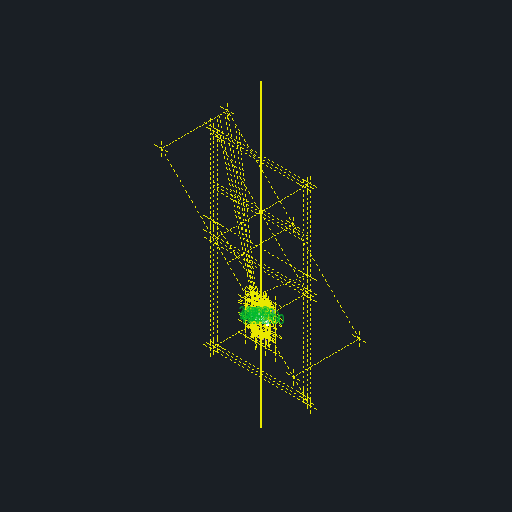
# Autodesk Inventor part: sensorbase
Saved by Autodesk Inventor 2023.5 (Build 275446000, 446)
## iProperties
Created: 2025-01-21
Part Number: sensorbase
Material: 一般
Document SubType Name: Modeling
Designer: IshiiLabHonda
Density: 1 g/cm^3
Appearance: 既定
Author: IshiiLabHonda
Autodesk Inventor part; units mm, degrees
ref_plane "YZ Plane" through (0, 0, 0) normal (1, 0, 0) x (0, 1, 0)
ref_plane "XZ Plane" through (0, 0, 0) normal (0, 1, 0) x (-1, 0, 0)
ref_plane "XY Plane" through (0, 0, 0) normal (0, 0, 1) x (1, 0, 0)
derived "chassis.ipt"
sketch "スケッチ1" plane through (0, 0, 0) normal (0, 0, 1) x (1, 0, 0)
  line L0 (-90, 90) -> (90, 90) construction
  line L1 (90, 90) -> (90, -90) construction
  line L2 (90, -90) -> (-90, -90) construction
  line L3 (-90, -90) -> (-90, 90) construction
  line L4 (-90, 90) -> (-90, 270) construction
  line L5 (-90, 270) -> (90, 270) construction
  line L6 (90, 270) -> (90, 90) construction
  line L7 (-90, 90) -> (90, -90) construction
  line L8 (90, 90) -> (-90, -90) construction
  line L9 (0, 0) -> (0, 10) construction
  line L10 (0, 0) -> (10, 0) construction
  line L11 (-90, 270) -> (90, 90) construction
  line L12 (-90, 90) -> (90, 270) construction
  line L13 (-96, 276) -> (96, 276) construction
  line L14 (96, 276) -> (96, -96) construction
  line L15 (96, -96) -> (-96, -96) construction
  line L16 (-96, -96) -> (-96, 276) construction
  line L17 (-84, 264) -> (84, 264) construction
  line L18 (84, 264) -> (84, -84) construction
  line L19 (84, -84) -> (-84, -84) construction
  line L20 (-84, -84) -> (-84, 264) construction
  line L21 (-96, 96) -> (96, 96) construction
  line L22 (-96, 84) -> (96, 84) construction
  line L23 (-63.6396, 63.6396) -> (63.6396, 190.9188) construction
  line L24 (63.6396, 190.9188) -> (190.9188, 63.6396) construction
  line L25 (190.9188, 63.6396) -> (63.6396, -63.6396) construction
  line L26 (63.6396, -63.6396) -> (-63.6396, 63.6396) construction
  line L27 (-190.9188, 190.9188) -> (-63.6396, 318.1981) construction
  line L28 (-63.6396, 318.1981) -> (63.6396, 190.9188) construction
  line L29 (-63.6396, 63.6396) -> (-190.9188, 190.9188) construction
  line L30 (-96, 120) -> (96, 120) construction
  line L31 (-96, 186) -> (96, 186) construction
  line L32 (-96, 174) -> (96, 174) construction
  line L33 (-96, 180) -> (96, 180) construction
  point P0 (-63.6396, 318.1981)
  point P1 (-90, 120)
  point P2 (90, 120)
  point P3 (0, 180)
sketch "スケッチ2" plane through (0, 0, 0) normal (0, 0, 1) x (1, 0, 0)
  line L0 (63.6396, 190.9188) -> (190.9188, 63.6396) construction
  line L1 (-63.6396, 318.1981) -> (63.6396, 190.9188) construction
  line L2 (-84, 264) -> (84, 264) construction
  line L3 (-90, 270) -> (90, 270) construction
  line L4 (90, 270) -> (90, 90) construction
  line L5 (-96, 276) -> (96, 276) construction
  line L6 (-90, 90) -> (90, 270) construction
  line L7 (-90, 270) -> (90, 90) construction
  line L8 (-63.6396, 63.6396) -> (63.6396, 190.9188) construction
  line L9 (-96, 120) -> (96, 120) construction
  line L10 (-90, 90) -> (90, 90) construction
  line L11 (-96, 96) -> (96, 96) construction
  line L12 (-96, 84) -> (96, 84) construction
  line L13 (90, -90) -> (-90, -90) construction
  line L14 (0, 0) -> (0, 10) construction
  line L15 (0, 0) -> (10, 0) construction
  line L16 (190.9188, 63.6396) -> (63.6396, -63.6396) construction
  line L17 (63.6396, -63.6396) -> (-63.6396, 63.6396) construction
  line L18 (84, -84) -> (-84, -84) construction
  line L19 (96, -96) -> (-96, -96) construction
  line L20 (-90, 90) -> (-90, 270) construction
  line L21 (-63.6396, 63.6396) -> (-190.9188, 190.9188) construction
  line L22 (-190.9188, 190.9188) -> (-63.6396, 318.1981) construction
  line L23 (96, 276) -> (96, -96) construction
  line L24 (-96, -96) -> (-96, 276) construction
  line L25 (84, 264) -> (84, -84) construction
  line L26 (-84, -84) -> (-84, 264) construction
  line L27 (90, 90) -> (90, -90) construction
  line L28 (-90, 90) -> (90, -90) construction
  line L29 (90, 90) -> (-90, -90) construction
  line L30 (-90, -90) -> (-90, 90) construction
  circle A0 centre (0, 0) radius 16.5 construction
  circle A1 centre (0, 0) radius 10 construction
  line L31 (20, 11.5) -> (28.75, 11.5) construction
  line L32 (28.75, 11.5) -> (28.75, -11.5) construction
  line L33 (28.75, -11.5) -> (20, -11.5) construction
  line L34 (20, -11.5) -> (20, 11.5) construction
  line L35 (20, 11.5) -> (18, 11.5) construction
  line L36 (18, 11.5) -> (18, -11.5) construction
  line L37 (18, -11.5) -> (20, -11.5) construction
  line L38 (18, 1.5) -> (17, 1.5) construction
  line L39 (17, -1.5) -> (18, -1.5) construction
  line L40 (-17, 24) -> (17, 24) construction
  line L41 (17, 24) -> (17, -24) construction
  line L42 (17, -24) -> (-17, -24) construction
  line L43 (-17, -24) -> (-17, 24) construction
  line L44 (-20, 11.5) -> (-18, 11.5) construction
  line L45 (-17, -1.5) -> (-18, -1.5) construction
  line L46 (-20, -11.5) -> (-20, 11.5) construction
  line L47 (-18, 11.5) -> (-18, -11.5) construction
  line L48 (-28.75, -11.5) -> (-20, -11.5) construction
  line L49 (-20, 11.5) -> (-28.75, 11.5) construction
  line L50 (-28.75, 11.5) -> (-28.75, -11.5) construction
  line L51 (-18, -11.5) -> (-20, -11.5) construction
  line L52 (-18, 1.5) -> (-17, 1.5) construction
  line L53 (-14.5, 24) -> (-14.5, -24) construction
  line L54 (14.5, 24) -> (14.5, -24) construction
  line L55 (-10.5, 24) -> (-10.5, 19) construction
  line L56 (-10.5, 19) -> (-14.5, 19) construction
  line L57 (-14.5, 24) -> (-10.5, 19) construction
  line L58 (-10.5, 24) -> (-14.5, 19) construction
  circle A2 centre (-12.5, 21.5) radius 1 construction
  line L59 (10.5, 24) -> (10.5, 19) construction
  line L60 (10.5, 19) -> (14.5, 19) construction
  line L61 (10.5, 24) -> (14.5, 19) construction
  line L62 (10.5, 19) -> (14.5, 24) construction
  circle A3 centre (12.5, 21.5) radius 1 construction
  line L63 (-14.5, -19) -> (-10.5, -19) construction
  line L64 (-10.5, -19) -> (-10.5, -24) construction
  line L65 (10.5, -24) -> (10.5, -19) construction
  line L66 (10.5, -19) -> (14.5, -19) construction
  line L67 (-14.5, -19) -> (-10.5, -24) construction
  line L68 (-10.5, -19) -> (-14.5, -24) construction
  circle A4 centre (-12.5, -21.5) radius 1 construction
  line L69 (10.5, -19) -> (14.5, -24) construction
  line L70 (14.5, -19) -> (10.5, -24) construction
  circle A5 centre (12.5, -21.5) radius 1 construction
  point P0 (90, 120)
  point P1 (-90, 120)
  point P2 (-63.6396, 318.1981)
  point P3 (-12.5, -21.5)
  point P4 (-12.5, 21.5)
sketch "スケッチ3" plane through (0, 0, 0) normal (0, 0, 1) x (1, 0, 0)
  line L0 (63.6396, 190.9188) -> (190.9188, 63.6396) construction
  line L1 (-63.6396, 318.1981) -> (63.6396, 190.9188) construction
  line L2 (-84, 264) -> (84, 264) construction
  line L3 (-90, 270) -> (90, 270) construction
  line L4 (90, 270) -> (90, 90) construction
  line L5 (-96, 276) -> (96, 276) construction
  line L6 (-90, 90) -> (90, 270) construction
  line L7 (-90, 270) -> (90, 90) construction
  line L8 (-63.6396, 63.6396) -> (63.6396, 190.9188) construction
  line L9 (-96, 120) -> (96, 120) construction
  line L10 (-90, 90) -> (90, 90) construction
  line L11 (-96, 96) -> (96, 96) construction
  line L12 (-96, 84) -> (96, 84) construction
  line L13 (90, -90) -> (-90, -90) construction
  line L14 (0, 0) -> (0, 10) construction
  line L15 (0, 0) -> (10, 0) construction
  line L16 (190.9188, 63.6396) -> (63.6396, -63.6396) construction
  line L17 (63.6396, -63.6396) -> (-63.6396, 63.6396) construction
  line L18 (84, -84) -> (-84, -84) construction
  line L19 (96, -96) -> (-96, -96) construction
  line L20 (-90, 90) -> (-90, 270) construction
  line L21 (-63.6396, 63.6396) -> (-190.9188, 190.9188) construction
  line L22 (-190.9188, 190.9188) -> (-63.6396, 318.1981) construction
  line L23 (96, 276) -> (96, -96) construction
  line L24 (-96, -96) -> (-96, 276) construction
  line L25 (84, 264) -> (84, -84) construction
  line L26 (-84, -84) -> (-84, 264) construction
  line L27 (90, 90) -> (90, -90) construction
  line L28 (-90, 90) -> (90, -90) construction
  line L29 (90, 90) -> (-90, -90) construction
  line L30 (-90, -90) -> (-90, 90) construction
  line L31 (-18, 1.5) -> (-17, 1.5) construction
  line L32 (-17, -1.5) -> (-18, -1.5) construction
  line L33 (-20, 11.5) -> (-18, 11.5) construction
  line L34 (-28.75, 11.5) -> (-28.75, -11.5) construction
  line L35 (63.6396, -63.6396) -> (-63.6396, 63.6396) construction
  line L36 (84, -84) -> (-84, -84) construction
  line L37 (-90, -90) -> (-90, 90) construction
  line L38 (96, -96) -> (-96, -96) construction
  line L39 (-90, 90) -> (90, 90) construction
  line L40 (90, -90) -> (-90, -90) construction
  line L41 (90, 90) -> (-90, -90) construction
  line L42 (-90, 90) -> (90, -90) construction
  line L43 (90, 90) -> (90, -90) construction
  line L44 (-28.75, -11.5) -> (-20, -11.5) construction
  line L45 (-20, 11.5) -> (-28.75, 11.5) construction
  line L46 (-18, 11.5) -> (-18, -11.5) construction
  line L47 (-18, -11.5) -> (-20, -11.5) construction
  line L48 (0, 0) -> (0, 10) construction
  line L49 (0, 0) -> (10, 0) construction
  circle A0 centre (0, 0) radius 16.5 construction
  circle A1 centre (0, 0) radius 10 construction
  line L50 (-14.5, 24) -> (-14.5, -24) construction
  line L51 (-17, 24) -> (17, 24) construction
  line L52 (-17, -24) -> (-17, 24) construction
  line L53 (17, -24) -> (-17, -24) construction
  line L54 (-14.5, -19) -> (-10.5, -19) construction
  circle A2 centre (-12.5, -21.5) radius 1 construction
  line L55 (-10.5, -19) -> (-14.5, -24) construction
  line L56 (-14.5, -19) -> (-10.5, -24) construction
  line L57 (-63.6396, 318.1981) -> (63.6396, 190.9188) construction
  line L58 (-84, 264) -> (84, 264) construction
  line L59 (-90, 270) -> (90, 270) construction
  line L60 (90, 270) -> (90, 90) construction
  line L61 (-96, 276) -> (96, 276) construction
  line L62 (-90, 90) -> (90, 270) construction
  line L63 (-90, 270) -> (90, 90) construction
  line L64 (-63.6396, 63.6396) -> (63.6396, 190.9188) construction
  line L65 (-96, 120) -> (96, 120) construction
  line L66 (-96, 96) -> (96, 96) construction
  line L67 (-96, 84) -> (96, 84) construction
  line L68 (84, 264) -> (84, -84) construction
  line L69 (96, 276) -> (96, -96) construction
  line L70 (-96, -96) -> (-96, 276) construction
  line L71 (-84, -84) -> (-84, 264) construction
  line L72 (-63.6396, 63.6396) -> (-190.9188, 190.9188) construction
  line L73 (-90, 90) -> (-90, 270) construction
  line L74 (-190.9188, 190.9188) -> (-63.6396, 318.1981) construction
  line L75 (-20, -11.5) -> (-20, 11.5) construction
  line L76 (10.5, -19) -> (14.5, -19) construction
  line L77 (10.5, -24) -> (10.5, -19) construction
  circle A3 centre (12.5, -21.5) radius 1 construction
  line L78 (10.5, -19) -> (14.5, -24) construction
  line L79 (14.5, -19) -> (10.5, -24) construction
  line L80 (-10.5, -19) -> (-10.5, -24) construction
  line L81 (63.6396, 190.9188) -> (190.9188, 63.6396) construction
  line L82 (190.9188, 63.6396) -> (63.6396, -63.6396) construction
  line L83 (20, 11.5) -> (28.75, 11.5) construction
  line L84 (28.75, 11.5) -> (28.75, -11.5) construction
  line L85 (17, -1.5) -> (18, -1.5) construction
  line L86 (18, -11.5) -> (20, -11.5) construction
  line L87 (28.75, -11.5) -> (20, -11.5) construction
  line L88 (14.5, 24) -> (14.5, -24) construction
  line L89 (17, 24) -> (17, -24) construction
  line L90 (18, 11.5) -> (18, -11.5) construction
  line L91 (20, -11.5) -> (20, 11.5) construction
  line L92 (20, 11.5) -> (18, 11.5) construction
  line L93 (18, 1.5) -> (17, 1.5) construction
  line L94 (-10.5, 24) -> (-10.5, 19) construction
  line L95 (10.5, 19) -> (14.5, 19) construction
  circle A4 centre (12.5, 21.5) radius 1 construction
  line L96 (10.5, 24) -> (14.5, 19) construction
  line L97 (10.5, 19) -> (14.5, 24) construction
  line L98 (10.5, 24) -> (10.5, 19) construction
  line L99 (-10.5, 19) -> (-14.5, 19) construction
  circle A5 centre (-12.5, 21.5) radius 1 construction
  line L100 (-14.5, 24) -> (-10.5, 19) construction
  line L101 (-10.5, 24) -> (-14.5, 19) construction
  line L102 (29.25, 41.5) -> (29.25, -41.5) construction
  line L103 (-29.25, -41.5) -> (-29.25, 41.5) construction
  line L104 (-29.25, 8.5) -> (-17, 8.5) construction
  line L105 (-17, 8.5) -> (-17, -8.5) construction
  line L106 (-17, -8.5) -> (-29.25, -8.5) construction
  line L107 (29.25, 8.5) -> (17, 8.5) construction
  line L108 (17, 8.5) -> (17, -8.5) construction
  line L109 (17, -8.5) -> (29.25, -8.5) construction
  line L110 (-2.7087, 12.8503) -> (-1.1893, 4.2332) construction
  line L111 (6.7279, 35.5721) -> (9.9419, 39.4023) construction
  line L112 (5.5106, 35.2882) -> (10.0101, 40.6505) construction
  line L113 (10.4899, 31.11) -> (5.5106, 35.2882) construction
  line L114 (10.0101, 40.6505) -> (10.4899, 31.11) construction
  line L115 (10.5581, 32.3582) -> (9.9419, 39.4023) construction
  line L116 (10.5581, 32.3582) -> (6.7279, 35.5721) construction
  line L117 (10.4899, 31.11) -> (12.788, 29.1817) construction
  line L118 (9.9419, 39.4023) -> (13.7721, 36.1884) construction
  line L119 (6.7279, 35.5721) -> (13.7721, 36.1884) construction
  line L120 (13.7721, 36.1884) -> (10.5581, 32.3582) construction
  line L121 (5.5106, 35.2882) -> (14.9894, 36.4724) construction
  line L122 (10.0101, 40.6505) -> (14.9894, 36.4724) construction
  line L123 (14.9894, 36.4724) -> (10.4899, 31.11) construction
  line L124 (12.788, 29.1817) -> (17.2875, 34.544) construction
  line L125 (17.2875, 34.544) -> (14.9894, 36.4724) construction
  line L126 (-3.5633, 11.938) -> (-2.695, 7.014) construction
  line L127 (-8.4873, 11.0698) -> (-2.695, 7.014) construction
  line L128 (-7.6191, 6.1457) -> (-3.5633, 11.938) construction
  line L129 (-9.1099, 11.7216) -> (-2.7087, 12.8503) construction
  line L130 (-7.6191, 6.1457) -> (-8.4873, 11.0698) construction
  line L131 (-1.1893, 4.2332) -> (-7.5905, 3.1045) construction
  line L132 (-63.6396, 318.1981) -> (-5.5912, 9.0419) construction
  line L133 (10.25, 35.8803) -> (-90, 120) construction
  line L134 (-5.5912, 9.0419) -> (-79.4589, 302.3788) construction
  line L135 (-5.5912, 9.0419) -> (-41.5175, 296.076) construction
  line L136 (-10.25, 35.8803) -> (90, 120) construction
  line L137 (-9.9419, 39.4023) -> (-6.7279, 35.5721) construction
  line L138 (-10.0101, 40.6505) -> (-5.5106, 35.2882) construction
  line L139 (-14.9894, 36.4724) -> (-10.0101, 40.6505) construction
  line L140 (-5.5106, 35.2882) -> (-14.9894, 36.4724) construction
  line L141 (-13.7721, 36.1884) -> (-6.7279, 35.5721) construction
  line L142 (-13.7721, 36.1884) -> (-9.9419, 39.4023) construction
  line L143 (-14.9894, 36.4724) -> (-17.2875, 34.544) construction
  line L144 (-6.7279, 35.5721) -> (-10.5581, 32.3582) construction
  line L145 (-9.9419, 39.4023) -> (-10.5581, 32.3582) construction
  line L146 (-10.0101, 40.6505) -> (-10.4899, 31.11) construction
  line L147 (-5.5106, 35.2882) -> (-10.4899, 31.11) construction
  line L148 (-10.4899, 31.11) -> (-14.9894, 36.4724) construction
  line L149 (-17.2875, 34.544) -> (-12.788, 29.1817) construction
  line L150 (-12.788, 29.1817) -> (-10.4899, 31.11) construction
  line L151 (-10.5581, 32.3582) -> (-13.7721, 36.1884) construction
  circle A6 centre (-7.0361, 32.05) radius 0.625 construction
  circle A7 centre (-7.0361, 32.05) radius 0.8 construction
  circle A8 centre (-7.0361, 32.05) radius 1.5 construction
  circle A9 centre (-16.0715, 34.6506) radius 1.5 construction
  circle A10 centre (-16.0715, 34.6506) radius 0.8 construction
  circle A11 centre (-16.0715, 34.6506) radius 0.625 construction
  line L152 (-2.695, 7.014) -> (-7.6191, 6.1457) construction
  line L153 (-7.9812, 5.3203) -> (-1.58, 6.449) construction
  line L154 (-8.0532, 8.6078) -> (-3.1291, 9.476) construction
  line L155 (-4.6361, 3.6254) -> (-5.157, 6.5799) construction
  line L156 (-8.4873, 11.0698) -> (-3.5633, 11.938) construction
  circle A12 centre (16.0715, 34.6506) radius 1.5 construction
  circle A13 centre (16.0715, 34.6506) radius 0.625 construction
  circle A14 centre (16.0715, 34.6506) radius 0.8 construction
  circle A15 centre (7.0361, 32.05) radius 1.5 construction
  circle A16 centre (7.0361, 32.05) radius 0.8 construction
  circle A17 centre (7.0361, 32.05) radius 0.625 construction
  line L157 (-29.25, -41.5) -> (29.25, -41.5) construction
  line L158 (-29.25, 41.5) -> (29.25, 41.5) construction
  line L159 (-10.25, 35.8803) -> (-7.0361, 32.05) construction
  line L160 (-29.25, 20.8653) -> (-13.3068, 41.5) construction
  line L161 (-29.25, -21.1569) -> (-8.9069, -41.5) construction
  line L162 (29.25, 20.8653) -> (13.3068, 41.5) construction
  line L163 (29.25, -21.1569) -> (8.9069, -41.5) construction
  line L164 (25.25, 19.5) -> (25.25, 14.5) construction
  line L165 (25.25, 14.5) -> (17, 14.5) construction
  line L166 (4.1128, 32.222) -> (-2.9985, 32.8014) construction
  line L167 (-17, 14.5) -> (-25.25, 14.5) construction
  line L168 (-25.25, 14.5) -> (-25.25, 19.5) construction
  line L169 (1.1893, 4.2332) -> (7.5905, 3.1045) construction
  line L170 (7.5905, 3.1045) -> (9.1099, 11.7216) construction
  line L171 (2.7087, 12.8503) -> (1.1893, 4.2332) construction
  line L172 (2.695, 7.014) -> (7.6191, 6.1457) construction
  line L173 (7.9812, 5.3203) -> (1.58, 6.449) construction
  line L174 (8.4873, 11.0698) -> (2.695, 7.014) construction
  line L175 (7.6191, 6.1457) -> (3.5633, 11.938) construction
  line L176 (3.5633, 11.938) -> (2.695, 7.014) construction
  line L177 (8.4873, 11.0698) -> (3.5633, 11.938) construction
  line L178 (7.6191, 6.1457) -> (8.4873, 11.0698) construction
  line L179 (9.1099, 11.7216) -> (2.7087, 12.8503) construction
  line L180 (-13.5, 30.3157) -> (-13.5, 24) construction
  line L181 (13.5, 30) -> (13.5, 24) construction
  line L182 (13.5, 24) -> (17, 24) construction
  line L183 (17, 24) -> (17, 14.5) construction
  line L184 (-13.5, 24) -> (-17, 24) construction
  line L185 (-17, 24) -> (-17, 14.5) construction
  line L186 (-13.5, 30.3157) -> (-2.9985, 32.8014) construction
  line L187 (13.5, 30) -> (4.1128, 32.222) construction
  line L188 (-17, -14.5) -> (-25.25, -14.5) construction
  line L189 (-25.25, -14.5) -> (-25.25, -19.5) construction
  line L190 (-25.25, -19.5) -> (-7.25, -37.5) construction
  line L191 (-7.25, -37.5) -> (7.25, -37.5) construction
  line L192 (7.25, -37.5) -> (25.25, -19.5) construction
  line L193 (25.25, -19.5) -> (25.25, -14.5) construction
  line L194 (25.25, -14.5) -> (17, -14.5) construction
  line L195 (17, -14.5) -> (17, -24) construction
  line L196 (17, -24) -> (13.5, -24) construction
  line L197 (13.5, -24) -> (11.356, -30.1704) construction
  line L198 (11.356, -30.1704) -> (-13.5, -30) construction
  line L199 (-13.5, -30) -> (-13.5, -24) construction
  line L200 (-13.5, -24) -> (-17, -24) construction
  line L201 (-17, -24) -> (-17, -14.5) construction
  line L202 (-9.1099, 11.7216) -> (-7.5905, 3.1045) construction
  line L203 (-9.4721, 10.8961) -> (-8.6039, 5.9721) construction
  line L204 (-14.3961, 10.0279) -> (-8.6039, 5.9721) construction
  line L205 (-13.5279, 5.1039) -> (-9.4721, 10.8961) construction
  line L206 (-13.5279, 5.1039) -> (-14.3961, 10.0279) construction
  line L207 (-7.5905, 3.1045) -> (-13.9918, 1.9758) construction
  line L208 (-14.3961, 10.0279) -> (-9.4721, 10.8961) construction
  line L209 (-13.962, 7.5659) -> (-9.038, 8.4341) construction
  line L210 (-8.6039, 5.9721) -> (-13.5279, 5.1039) construction
  line L211 (-10.5449, 2.5836) -> (-11.0659, 5.538) construction
  line L212 (-15.5112, 10.5929) -> (-9.1099, 11.7216) construction
  line L213 (9.4721, 10.8961) -> (8.6039, 5.9721) construction
  line L214 (9.1099, 11.7216) -> (7.5905, 3.1045) construction
  line L215 (14.3961, 10.0279) -> (9.4721, 10.8961) construction
  line L216 (13.962, 7.5659) -> (9.038, 8.4341) construction
  line L217 (10.5449, 2.5836) -> (11.0659, 5.538) construction
  line L218 (15.5112, 10.5929) -> (9.1099, 11.7216) construction
  line L219 (13.5279, 5.1039) -> (9.4721, 10.8961) construction
  line L220 (8.6039, 5.9721) -> (13.5279, 5.1039) construction
  line L221 (14.3961, 10.0279) -> (8.6039, 5.9721) construction
  line L222 (13.5279, 5.1039) -> (14.3961, 10.0279) construction
  line L223 (13.9918, 1.9758) -> (15.5112, 10.5929) construction
  line L224 (7.5905, 3.1045) -> (13.9918, 1.9758) construction
  line L225 (-25.25, 19.5) -> (-11.3425, 37.5) construction
  line L226 (-11.3425, 37.5) -> (11.3425, 37.5) construction
  line L227 (11.3425, 37.5) -> (25.25, 19.5) construction
  circle A18 centre (0, 0) radius 4.25 construction
  line L228 (-11.5, 8) -> (-68.7791, 313.0586) construction
  line L229 (-11.5, 8) -> (-84.3887, 297.449) construction
  line L230 (-11.5, 8) -> (-48.4208, 302.9793) construction
  line L231 (-15.5112, 10.5929) -> (-13.9918, 1.9758) construction
  line L232 (-14.3825, 4.1916) -> (-7.9812, 5.3203) construction
  circle A19 centre (-10.5, -27) radius 1
  circle A20 centre (10.5, 27) radius 1
  circle A21 centre (10.5, 27) radius 2
  circle A22 centre (-10.5, -27) radius 2
  circle A23 centre (0, -27) radius 1
  circle A24 centre (0, -27) radius 2
  circle A25 centre (0, 27) radius 1
  circle A26 centre (0, 27) radius 2
  line L233 (0, 27) -> (10.5, 27) construction
  line L234 (-10.5, -27) -> (0, -27) construction
  line L235 (13.5, 30) -> (-3, 30)
  line L236 (-3, 30) -> (-3, 24)
  line L237 (-13.5, 24) -> (-3, 24)
  line L238 (-13.5, -30) -> (3, -30)
  line L239 (3, -30) -> (3, -24)
  line L240 (3, -24) -> (13.5, -24)
  line L241 (-16.1606, 31.2641) -> (-6.1594, 29.9135)
  line L242 (-6.1594, 29.9135) -> (-5.0634, 31.332)
  line L243 (-5.0634, 31.332) -> (-4.8147, 37.5)
  line L244 (6.1594, 29.9135) -> (5.0634, 31.332)
  line L245 (16.1606, 31.2641) -> (6.1594, 29.9135)
  line L246 (5.0634, 31.332) -> (4.8147, 37.5)
  line L247 (-10.5, -27) -> (-14.125, -30.625) construction
  line L248 (-15.5392, -29.2108) -> (-13.5, -24)
  line L249 (-12.7108, -32.0392) -> (-7.5, -30)
  line L250 (10.5, 27) -> (13.5, 30) construction
  line L251 (16.1606, 31.2641) -> (10.0926, 30)
  line L252 (-10.5, -19) -> (-10.5, -20.4081)
  line L253 (-10.5, -20.4081) -> (-7.5, -21.5)
  line L254 (-7.5, -21.5) -> (7.5, -21.5)
  line L255 (7.5, -21.5) -> (10.5, -20.4081)
  line L256 (10.5, -20.4081) -> (10.5, -19)
  line L257 (10.5, -19) -> (-10.5, -19)
  line L258 (7.5, 21.5) -> (10.5, 20.4081)
  line L259 (10.5, 20.4081) -> (10.5, 19)
  line L260 (-7.5, 21.5) -> (7.5, 21.5)
  line L261 (10.5, 19) -> (-10.5, 19)
  line L262 (-10.5, 19) -> (-10.5, 20.4081)
  line L263 (-10.5, 20.4081) -> (-7.5, 21.5)
  line L264 (-5.3602, -19) -> (-14.5, -13.3971)
  line L265 (-14.5, -13.3971) -> (-14.5, -15.3971)
  line L266 (0, 0) -> (-9.9301, -16.1985) construction
  line L267 (14.5, -13.3971) -> (14.5, -15.3971)
  line L268 (5.3602, -19) -> (14.5, -13.3971)
  line L269 (-5.3602, 19) -> (-14.5, 13.3971)
  line L270 (-14.5, 13.3971) -> (-14.5, 15.3971)
  line L271 (5.3602, 19) -> (14.5, 13.3971)
  line L272 (14.5, 13.3971) -> (14.5, 15.3971)
  line L273 (-14.5, -15.3971) -> (-10.5, -20.4081)
  line L274 (10.5, -20.4081) -> (14.5, -15.3971)
  line L275 (-14.5, 15.3971) -> (-10.5, 20.4081)
  line L276 (14.5, 15.3971) -> (10.5, 20.4081)
  line L277 (-5.3602, -19) -> (-9.4462, -17.5128)
  line L278 (-9.4462, -17.5128) -> (-14.5, -13.3971)
  line L279 (-10.5, -20.4081) -> (-9.4462, -17.5128) construction
  line L280 (9.4462, -17.5128) -> (14.5, -13.3971)
  line L281 (5.3602, -19) -> (9.4462, -17.5128)
  line L282 (-5.3602, 19) -> (-9.4462, 17.5128)
  line L283 (-9.4462, 17.5128) -> (-14.5, 13.3971)
  line L284 (9.4462, 17.5128) -> (14.5, 13.3971)
  line L285 (5.3602, 19) -> (9.4462, 17.5128)
  point P0 (90, 120)
  point P1 (90, 120)
  point P2 (25.25, 25.1515)
  point P3 (11.5, 8)
  point P4 (11.5, 8)
  point P5 (-5.5912, 9.0419)
  point P6 (-5.5912, 9.0419)
  point P7 (13.6038, 24)
  point P8 (6.0926, 30)
sketch "スケッチ4" plane through (0, 0, 0) normal (1, 0, 0) x (0, 1, 0)
  circle A0 centre (15.0669, 9.7) radius 4.35 construction
  line L0 (0, 8.7) -> (0, 9.7) construction
  circle A1 centre (0, 8.7) radius 10.65 construction
  circle A2 centre (0, 8.7) radius 11.5 construction
  line L1 (-25, -2.8) -> (25, -2.8) construction
  line L2 (-25, -1) -> (25, -1) construction
  line L3 (-25, 0) -> (25, 0) construction
  line L4 (0, 8.7) -> (1, 8.7) construction
  circle A3 centre (-13, 8.7) radius 2.25 construction
  line L5 (0, -7.4) -> (0, 24.8)
  line L6 (-178.8396, 0) -> (401.0377, 0)
  point P0 (0, 0)
  point P1 (0, 0)
sketch "スケッチ5" plane through (0, 0, 0) normal (0, 0, 1) x (1, 0, 0)
  line L0 (0, 0) -> (0, 10) construction
  line L1 (0, 0) -> (10, 0) construction
  line L2 (-17, -1.5) -> (-18, -1.5) construction
  line L3 (-28.75, -11.5) -> (-20, -11.5) construction
  line L4 (-18, 1.5) -> (-17, 1.5) construction
  line L5 (-18, 11.5) -> (-18, -11.5) construction
  line L6 (-20, 11.5) -> (-18, 11.5) construction
  line L7 (-20, -11.5) -> (-20, 11.5) construction
  line L8 (-20, 11.5) -> (-28.75, 11.5) construction
  line L9 (-28.75, 11.5) -> (-28.75, -11.5) construction
  line L10 (28.75, 11.5) -> (28.75, -11.5) construction
  line L11 (28.75, -11.5) -> (20, -11.5) construction
  line L12 (20, 11.5) -> (28.75, 11.5) construction
  line L13 (20, 11.5) -> (18, 11.5) construction
  line L14 (18, 1.5) -> (17, 1.5) construction
  line L15 (20, -11.5) -> (20, 11.5) construction
  line L16 (18, -11.5) -> (20, -11.5) construction
  line L17 (18, 11.5) -> (18, -11.5) construction
  circle A0 centre (0, 0) radius 10 construction
  line L18 (17, 24) -> (17, -24) construction
  line L19 (-17, 24) -> (17, 24) construction
  line L20 (14.5, 24) -> (14.5, -24) construction
  circle A1 centre (0, 0) radius 16.5 construction
  line L21 (-14.5, 24) -> (-14.5, -24) construction
  line L22 (-17, -24) -> (-17, 24) construction
  line L23 (17, -24) -> (-17, -24) construction
  line L24 (17, -1.5) -> (18, -1.5) construction
  line L25 (-18, -11.5) -> (-20, -11.5) construction
  line L26 (-10.5, 19) -> (-14.5, 19) construction
  line L27 (-10.5, 24) -> (-10.5, 19) construction
  circle A2 centre (-12.5, 21.5) radius 1 construction
  line L28 (-14.5, 24) -> (-10.5, 19) construction
  line L29 (-10.5, 24) -> (-14.5, 19) construction
  line L30 (10.5, 24) -> (10.5, 19) construction
  circle A3 centre (12.5, 21.5) radius 1 construction
  line L31 (10.5, 24) -> (14.5, 19) construction
  line L32 (10.5, 19) -> (14.5, 24) construction
  line L33 (10.5, 19) -> (14.5, 19) construction
  line L34 (-14.5, -19) -> (-10.5, -19) construction
  circle A4 centre (-12.5, -21.5) radius 1 construction
  line L35 (-14.5, -19) -> (-10.5, -24) construction
  line L36 (-10.5, -19) -> (-14.5, -24) construction
  line L37 (-10.5, -19) -> (-10.5, -24) construction
  line L38 (10.5, -19) -> (14.5, -19) construction
  circle A5 centre (12.5, -21.5) radius 1 construction
  line L39 (10.5, -19) -> (14.5, -24) construction
  line L40 (14.5, -19) -> (10.5, -24) construction
  line L41 (10.5, -24) -> (10.5, -19) construction
  line L42 (13.5, 24) -> (17, 24) construction
  line L43 (4.1128, 32.222) -> (-2.9985, 32.8014) construction
  line L44 (17, 8.5) -> (17, -8.5) construction
  line L45 (10.5449, 2.5836) -> (11.0659, 5.538) construction
  line L46 (13.5279, 5.1039) -> (9.4721, 10.8961) construction
  line L47 (8.6039, 5.9721) -> (13.5279, 5.1039) construction
  line L48 (13.962, 7.5659) -> (9.038, 8.4341) construction
  line L49 (14.3961, 10.0279) -> (9.4721, 10.8961) construction
  line L50 (14.3961, 10.0279) -> (8.6039, 5.9721) construction
  line L51 (13.5279, 5.1039) -> (14.3961, 10.0279) construction
  line L52 (7.5905, 3.1045) -> (13.9918, 1.9758) construction
  line L53 (15.5112, 10.5929) -> (9.1099, 11.7216) construction
  line L54 (13.9918, 1.9758) -> (15.5112, 10.5929) construction
  line L55 (20, 11.5) -> (28.75, 11.5) construction
  line L56 (20, 11.5) -> (18, 11.5) construction
  line L57 (10.5, 19) -> (14.5, 19) construction
  circle A6 centre (12.5, 21.5) radius 1 construction
  line L58 (29.25, 8.5) -> (17, 8.5) construction
  line L59 (13.5, 30) -> (13.5, 24) construction
  line L60 (25.25, 14.5) -> (17, 14.5) construction
  line L61 (25.25, 19.5) -> (25.25, 14.5) construction
  line L62 (13.5, 30) -> (4.1128, 32.222) construction
  line L63 (17, 24) -> (17, 14.5) construction
  line L64 (9.1099, 11.7216) -> (2.7087, 12.8503) construction
  line L65 (8.4873, 11.0698) -> (3.5633, 11.938) construction
  line L66 (-8.4873, 11.0698) -> (-3.5633, 11.938) construction
  line L67 (-17, 8.5) -> (-17, -8.5) construction
  line L68 (-7.6191, 6.1457) -> (-8.4873, 11.0698) construction
  line L69 (-7.5905, 3.1045) -> (-13.9918, 1.9758) construction
  line L70 (-14.3825, 4.1916) -> (-7.9812, 5.3203) construction
  line L71 (-10.5449, 2.5836) -> (-11.0659, 5.538) construction
  line L72 (-8.6039, 5.9721) -> (-13.5279, 5.1039) construction
  line L73 (-13.962, 7.5659) -> (-9.038, 8.4341) construction
  line L74 (-14.3961, 10.0279) -> (-8.6039, 5.9721) construction
  line L75 (-13.5279, 5.1039) -> (-14.3961, 10.0279) construction
  line L76 (-15.5112, 10.5929) -> (-13.9918, 1.9758) construction
  line L77 (-9.4721, 10.8961) -> (-8.6039, 5.9721) construction
  line L78 (-13.5279, 5.1039) -> (-9.4721, 10.8961) construction
  line L79 (-9.1099, 11.7216) -> (-7.5905, 3.1045) construction
  line L80 (-14.3961, 10.0279) -> (-9.4721, 10.8961) construction
  line L81 (-15.5112, 10.5929) -> (-9.1099, 11.7216) construction
  line L82 (2.7087, 12.8503) -> (1.1893, 4.2332) construction
  line L83 (3.5633, 11.938) -> (2.695, 7.014) construction
  line L84 (7.6191, 6.1457) -> (3.5633, 11.938) construction
  line L85 (7.6191, 6.1457) -> (8.4873, 11.0698) construction
  line L86 (2.695, 7.014) -> (7.6191, 6.1457) construction
  line L87 (9.4721, 10.8961) -> (8.6039, 5.9721) construction
  line L88 (7.9812, 5.3203) -> (1.58, 6.449) construction
  line L89 (1.1893, 4.2332) -> (7.5905, 3.1045) construction
  line L90 (7.5905, 3.1045) -> (9.1099, 11.7216) construction
  line L91 (9.1099, 11.7216) -> (7.5905, 3.1045) construction
  line L92 (8.4873, 11.0698) -> (2.695, 7.014) construction
  line L93 (0, 0) -> (0, 10) construction
  circle A7 centre (0, 0) radius 4.25 construction
  line L94 (-2.7087, 12.8503) -> (-1.1893, 4.2332) construction
  line L95 (-3.5633, 11.938) -> (-2.695, 7.014) construction
  line L96 (-4.6361, 3.6254) -> (-5.157, 6.5799) construction
  line L97 (-1.1893, 4.2332) -> (-7.5905, 3.1045) construction
  line L98 (-2.695, 7.014) -> (-7.6191, 6.1457) construction
  line L99 (-7.6191, 6.1457) -> (-3.5633, 11.938) construction
  line L100 (-8.4873, 11.0698) -> (-2.695, 7.014) construction
  line L101 (-7.9812, 5.3203) -> (-1.58, 6.449) construction
  line L102 (-11.3425, 37.5) -> (11.3425, 37.5) construction
  line L103 (-10.25, 35.8803) -> (-7.0361, 32.05) construction
  line L104 (11.3425, 37.5) -> (25.25, 19.5) construction
  line L105 (29.25, 20.8653) -> (13.3068, 41.5) construction
  circle A8 centre (16.0715, 34.6506) radius 1.5 construction
  circle A9 centre (16.0715, 34.6506) radius 0.8 construction
  circle A10 centre (16.0715, 34.6506) radius 0.625 construction
  line L106 (0, 0) -> (0, 10) construction
  line L107 (0, 0) -> (10, 0) construction
  circle A11 centre (0, 0) radius 16.5 construction
  circle A12 centre (0, 0) radius 10 construction
  line L108 (-14.5, 24) -> (-14.5, -24) construction
  line L109 (-17, 24) -> (17, 24) construction
  line L110 (-9.1099, 11.7216) -> (-2.7087, 12.8503) construction
  line L111 (-14.5, -19) -> (-10.5, -19) construction
  circle A13 centre (-12.5, -21.5) radius 1 construction
  line L112 (-17, -24) -> (-17, 24) construction
  line L113 (17, -24) -> (-17, -24) construction
  line L114 (-10.5, -19) -> (-14.5, -24) construction
  line L115 (-14.5, -19) -> (-10.5, -24) construction
  line L116 (-28.75, 11.5) -> (-28.75, -11.5) construction
  line L117 (-9.9419, 39.4023) -> (-6.7279, 35.5721) construction
  line L118 (-10.0101, 40.6505) -> (-5.5106, 35.2882) construction
  line L119 (-13.7721, 36.1884) -> (-6.7279, 35.5721) construction
  line L120 (-5.5106, 35.2882) -> (-14.9894, 36.4724) construction
  line L121 (-13.7721, 36.1884) -> (-9.9419, 39.4023) construction
  line L122 (-14.9894, 36.4724) -> (-10.0101, 40.6505) construction
  line L123 (-14.9894, 36.4724) -> (-17.2875, 34.544) construction
  circle A14 centre (-7.0361, 32.05) radius 0.625 construction
  circle A15 centre (-7.0361, 32.05) radius 0.8 construction
  circle A16 centre (-7.0361, 32.05) radius 1.5 construction
  line L124 (-5.5106, 35.2882) -> (-10.4899, 31.11) construction
  line L125 (-6.7279, 35.5721) -> (-10.5581, 32.3582) construction
  line L126 (-9.9419, 39.4023) -> (-10.5581, 32.3582) construction
  line L127 (-10.0101, 40.6505) -> (-10.4899, 31.11) construction
  line L128 (-12.788, 29.1817) -> (-10.4899, 31.11) construction
  line L129 (-10.5581, 32.3582) -> (-13.7721, 36.1884) construction
  circle A17 centre (-16.0715, 34.6506) radius 0.625 construction
  circle A18 centre (-16.0715, 34.6506) radius 0.8 construction
  circle A19 centre (-16.0715, 34.6506) radius 1.5 construction
  line L130 (-17.2875, 34.544) -> (-12.788, 29.1817) construction
  line L131 (-10.4899, 31.11) -> (-14.9894, 36.4724) construction
  line L132 (-18, 11.5) -> (-18, -11.5) construction
  line L133 (-20, 11.5) -> (-18, 11.5) construction
  line L134 (-10.5, 24) -> (-10.5, 19) construction
  line L135 (-10.5, 19) -> (-14.5, 19) construction
  circle A20 centre (-12.5, 21.5) radius 1 construction
  line L136 (-14.5, 24) -> (-10.5, 19) construction
  line L137 (-10.5, 24) -> (-14.5, 19) construction
  line L138 (-8.0532, 8.6078) -> (-3.1291, 9.476) construction
  line L139 (-17, 14.5) -> (-25.25, 14.5) construction
  line L140 (-25.25, 14.5) -> (-25.25, 19.5) construction
  line L141 (-13.5, 30.3157) -> (-2.9985, 32.8014) construction
  line L142 (-13.5, 30.3157) -> (-13.5, 24) construction
  line L143 (-13.5, 24) -> (-17, 24) construction
  line L144 (-25.25, 19.5) -> (-11.3425, 37.5) construction
  line L145 (-17, 24) -> (-17, 14.5) construction
  line L146 (-17, -24) -> (-17, -14.5) construction
  line L147 (-17, -14.5) -> (-25.25, -14.5) construction
  line L148 (-25.25, -14.5) -> (-25.25, -19.5) construction
  line L149 (-25.25, -19.5) -> (-7.25, -37.5) construction
  line L150 (-29.25, -21.1569) -> (-8.9069, -41.5) construction
  line L151 (10.5, -19) -> (14.5, -19) construction
  line L152 (10.5, -24) -> (10.5, -19) construction
  circle A21 centre (12.5, -21.5) radius 1 construction
  line L153 (10.5, -19) -> (14.5, -24) construction
  line L154 (14.5, -19) -> (10.5, -24) construction
  line L155 (-10.5, -19) -> (-10.5, -24) construction
  line L156 (18, -11.5) -> (20, -11.5) construction
  line L157 (28.75, -11.5) -> (20, -11.5) construction
  line L158 (17, -8.5) -> (29.25, -8.5) construction
  line L159 (-29.25, -41.5) -> (29.25, -41.5) construction
  line L160 (-7.25, -37.5) -> (7.25, -37.5) construction
  line L161 (11.356, -30.1704) -> (-13.5, -30) construction
  line L162 (13.5, -24) -> (11.356, -30.1704) construction
  line L163 (17, -24) -> (13.5, -24) construction
  line L164 (17, -14.5) -> (17, -24) construction
  line L165 (7.25, -37.5) -> (25.25, -19.5) construction
  line L166 (29.25, -21.1569) -> (8.9069, -41.5) construction
  line L167 (25.25, -14.5) -> (17, -14.5) construction
  line L168 (25.25, -19.5) -> (25.25, -14.5) construction
  line L169 (10.0101, 40.6505) -> (14.9894, 36.4724) construction
  line L170 (10.4899, 31.11) -> (12.788, 29.1817) construction
  line L171 (12.788, 29.1817) -> (17.2875, 34.544) construction
  line L172 (17.2875, 34.544) -> (14.9894, 36.4724) construction
  line L173 (-29.25, 41.5) -> (29.25, 41.5) construction
  line L174 (13.7721, 36.1884) -> (10.5581, 32.3582) construction
  line L175 (14.9894, 36.4724) -> (10.4899, 31.11) construction
  circle A22 centre (7.0361, 32.05) radius 0.625 construction
  circle A23 centre (7.0361, 32.05) radius 0.8 construction
  line L176 (10.5581, 32.3582) -> (9.9419, 39.4023) construction
  line L177 (9.9419, 39.4023) -> (13.7721, 36.1884) construction
  circle A24 centre (7.0361, 32.05) radius 1.5 construction
  line L178 (10.5581, 32.3582) -> (6.7279, 35.5721) construction
  line L179 (6.7279, 35.5721) -> (13.7721, 36.1884) construction
  line L180 (5.5106, 35.2882) -> (14.9894, 36.4724) construction
  line L181 (10.0101, 40.6505) -> (10.4899, 31.11) construction
  line L182 (6.7279, 35.5721) -> (9.9419, 39.4023) construction
  line L183 (5.5106, 35.2882) -> (10.0101, 40.6505) construction
  line L184 (10.4899, 31.11) -> (5.5106, 35.2882) construction
  line L185 (-13.5, -24) -> (-17, -24) construction
  line L186 (-13.5, -30) -> (-13.5, -24) construction
  line L187 (-17, -8.5) -> (-29.25, -8.5) construction
  line L188 (-20, -11.5) -> (-20, 11.5) construction
  line L189 (17, -1.5) -> (18, -1.5) construction
  line L190 (18, 1.5) -> (17, 1.5) construction
  line L191 (-29.25, -41.5) -> (-29.25, 41.5) construction
  line L192 (18, 11.5) -> (18, -11.5) construction
  line L193 (20, -11.5) -> (20, 11.5) construction
  line L194 (29.25, 41.5) -> (29.25, -41.5) construction
  line L195 (28.75, 11.5) -> (28.75, -11.5) construction
  line L196 (14.5, 24) -> (14.5, -24) construction
  line L197 (17, 24) -> (17, -24) construction
  line L198 (10.5, 24) -> (14.5, 19) construction
  line L199 (10.5, 19) -> (14.5, 24) construction
  line L200 (10.5, 24) -> (10.5, 19) construction
  line L201 (-20, 11.5) -> (-28.75, 11.5) construction
  line L202 (-28.75, -11.5) -> (-20, -11.5) construction
  line L203 (-18, -11.5) -> (-20, -11.5) construction
  line L204 (-18, 1.5) -> (-17, 1.5) construction
  line L205 (-17, -1.5) -> (-18, -1.5) construction
  line L206 (0, 0) -> (10, 0) construction
  line L207 (-29.25, 20.8653) -> (-13.3068, 41.5) construction
  line L208 (-29.25, 8.5) -> (-17, 8.5) construction
  line L209 (0, 0) -> (0, 10) construction
  line L210 (0, 0) -> (10, 0) construction
  line L211 (0, -10.65) -> (0, 10.65) construction
  line L212 (0, 0) -> (0, 1) construction
  line L213 (0, -15.25) -> (0, -10.75) construction
  line L214 (0, 10.7169) -> (0, 19.4169) construction
  line L215 (0, -11.5) -> (0, 11.5) construction
  line L216 (0, -25) -> (0, 25) construction
  line L217 (0, -25) -> (0, 25) construction
  line L218 (0, -25) -> (0, 25) construction
  circle A25 centre (-12.5, 6) radius 1
  circle A26 centre (-12.5, 6) radius 2.5
  circle A27 centre (-12.5, 6) radius 0.8 construction
  circle A28 centre (12.5, 6) radius 1
  circle A29 centre (12.5, 6) radius 2.5
  circle A30 centre (12.5, 6) radius 0.8 construction
  line L219 (-12.5, 3.5) -> (12.5, 3.5)
  line L220 (-12.5, 8.5) -> (12.5, 8.5)
  line L221 (-3.499, 11) -> (3.499, 11)
  line L222 (3.499, 11) -> (13.147, 8.4148)
  line L223 (-13.147, 8.4148) -> (-3.499, 11)
  line L224 (-10.088, 3.5) -> (0, 5.6443)
  line L225 (0, 5.6443) -> (10.088, 3.5)
  line L226 (-1.8, 11) -> (0, 10.3449)
  line L227 (0, 10.3449) -> (1.8, 11)
  circle A31 centre (0, 7.7213) radius 0.8
  circle A32 centre (0, 7.7213) radius 1.5
  circle A33 centre (-14.75, 0.7) radius 0.8
  circle A34 centre (-14.75, 0.7) radius 1.5
  circle A35 centre (14.75, 0.7) radius 0.8
  circle A36 centre (14.75, 0.7) radius 1.5
  line L228 (-10.088, 3.5) -> (-13.653, -0.323)
  line L229 (10.088, 3.5) -> (13.653, -0.323)
  line L230 (14.9359, 6.5624) -> (16.2115, 1.0375)
  line L231 (-14.9359, 6.5624) -> (-16.2115, 1.0375)
  line L232 (-14.9445, 6.5254) -> (-13.0214, 8.4485)
  line L233 (14.9445, 6.5254) -> (13.0214, 8.4485)
  circle A37 centre (-7.25, 0) radius 0.8
  circle A38 centre (-7.25, 0) radius 1.5
  line L234 (-11.0158, 2.505) -> (-8.448, -0.9027)
  line L235 (-5.7776, -0.2862) -> (-4.8241, 4.6189)
  circle A39 centre (7.25, 0) radius 0.8
  circle A40 centre (7.25, 0) radius 1.5
  line L236 (11.0158, 2.505) -> (8.448, -0.9027)
  line L237 (5.7776, -0.2862) -> (4.8241, 4.6189)
  circle A41 centre (0, 0) radius 5.75 construction
  point P0 (-12.5, 21.5)
  point P1 (-12.5, -21.5)
  point P2 (25.25, 25.1515)
  point P3 (11.5, 8)
  point P4 (11.5, 8)
  point P5 (-11.5, 8)
  point P6 (-11.5, 8)
  point P7 (-5.5912, 9.0419)
  point P8 (-5.5912, 9.0419)
  point P9 (-5.5912, 9.0419)
  point P10 (10.25, 35.8803)
  point P11 (0, -13)
  point P12 (0, 15.0669)
  point P13 (4.6195, 3.5)
  point P14 (7.1992, 3.5)
  point P15 (-7.1992, 3.5)
  point P16 (-4.6195, 3.5)
  point P17 (13.0258, 8.4441)
  point P18 (14.9441, 6.5258)
  point P19 (-14.9441, 6.5258)
  point P20 (-13.0258, 8.4441)
  point P21 (14.9445, 6.5254)
  point P22 (13.0214, 8.4485)
  point P23 (11.0158, 2.505)
  point P24 (4.8241, 4.6189)
  dimension "d1" = 2
  dimension "d2" = 6
  dimension "d3" = 2
  dimension "d4" = 1.6
  dimension "d5" = 5
  dimension "d7" = 2.5
  dimension "d8" = 15
  dimension "d9" = 1.6
  dimension "d10" = 3
  dimension "d11" = 1.6
  dimension "d12" = 3
  dimension "d19" = 0.7
  dimension "d20" = 0.25
  dimension "d21" = 4.7006
  dimension "d22" = 12
  dimension "d23" = 47
  dimension "d24" = 12
  dimension "d25" = 20
  dimension "d26" = 3.6
  dimension "d28" = 30
  dimension "d29" = 2.1
  dimension "d34" = 1.6
  dimension "d35" = 3
  dimension "d36" = 20
  dimension "d38" = 80
  dimension "d42" = 11.5
  dimension "d43" = 4.2213
  dimension "d44" = 113
  constraints: 38 end point, 17 centre point, 16 point on circle, 15 horizontal alignment, 15 tangent, 10 coincident, 8 point on line, 7 equal radius, 1 horizontal, 29 other
  measures "d1" distance from line of L21 A25.centre
  measures "d3" diameter of A25
  measures "d4" diameter of A27
  measures "d5" diameter of A26
  measures "d7" distance between parallel lines of L220 L221
  measures "d8" angle of L220 L223
  measures "d9" diameter of A31
  measures "d10" diameter of A32
  measures "d11" diameter of A33
  measures "d12" diameter of A34
  measures "d20" distance from line of A34.centre L21
  measures "d21" distance of L224.end L226.end
  measures "d22" angle of L219 L224
  measures "d23" angle of L219 L228
  measures "d24" angle of L219 L225
  measures "d25" angle of L226 L221
  measures "d26" distance of L227.end L226.start
  measures "d28" angle of L232 L223
  measures "d29" distance from line of L232 A26.centre
  measures "d34" diameter of A37
  measures "d35" diameter of A38
  measures "d36" diameter of A0
  measures "d38" angle of L228 L234
  measures "d42" diameter of A41
  measures "d43" distance from line of L219 A31.centre
  measures "d44" angle of L224 L235
extrude "押し出し1" add sketch "スケッチ5" against normal blind 1 contours A25 | A26 L232 | A26 L220 A32 A29 L219 L225 L224 | A26 L232 L223 L221 L226 L227 L222 L233 A29 L220 A32 | L219 L228 A34 L231 A26 | L232 A26 | A26 L223 L232 | A32 L220 A31 | L220 A31 A32 | L224 L235 L219 | A31 L220 | L220 A31 | A34 | L235 L224 L225 L237 L219 | A29 L233 | L237 L225 L219 | L221 L227 L226 | A29 L230 A36 L229 L219 | L233 L222 A29 | A29 L233 | A36 | A28
extrude "押し出し2" cut sketch "スケッチ5" against normal blind 1 contours A25 | A31 L220 | L220 A31 | L221 L227 L226 | A28 | A33 | A35
extrude "押し出し3" cut sketch "スケッチ5" against normal blind 1 contours L224 L235 L219 | L235 L224 L225 L237 L219 | L237 L225 L219
extrude "押し出し4" cut sketch "スケッチ5" against normal blind 1 contours L232 A26 | A29 L233 picked at (-14.1889, 7.4908) picked at (14.2419, 7.3514)
extrude "押し出し5" cut sketch "スケッチ5" against normal blind 1 contours A26 L223 L232 | L233 L222 A29
extrude "押し出し6" add sketch "スケッチ5" against normal blind 1 contours L224 L235 L219 | L219 L235 A38 L234 L228 | L237 L225 L219 | L219 L229 L236 A40 L237 | A38 | A40
fillet "フィレット1" radius 0.75 9 edges at (-11.0158, 2.505, -0.5) (-4.8241, 4.6189, -0.5) (4.8241, 4.6189, -0.5) (11.0158, 2.505, -0.5) (3.499, 11, -0.5) (1.8, 11, -0.5) (0, 10.3449, -0.5) (-1.8, 11, -0.5) (0, 5.6443, -0.5)
